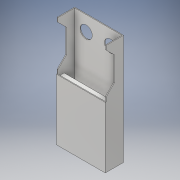
# Autodesk Inventor part: USB_Contact
Saved by Autodesk Inventor 2018 (Build 220112000, 112)
## iProperties
Created: 2018-02-01
Part Number: USB_Contact
Material: Generic
Document SubType Name: Modeling
Designer: Mandus
Density: 1 g/cm^3
Appearance: Default
Author: Mandus
Autodesk Inventor part; units mm, degrees
ref_plane "YZ Plane" through (0, 0, 0) normal (1, 0, 0) x (0, 1, 0)
ref_plane "XZ Plane" through (0, 0, 0) normal (0, 1, 0) x (-1, 0, 0)
ref_plane "XY Plane" through (0, 0, 0) normal (0, 0, 1) x (1, 0, 0)
sketch "Sketch1" plane through (0, 0, 0) normal (0, 1, 0) x (-1, 0, 0)
  line L0 (5.3848, 9.7652) -> (-6.6152, 9.7652)
  line L1 (-6.6152, 9.7652) -> (-6.6152, 5.2652)
  line L2 (-6.6152, 5.2652) -> (5.3848, 5.2652)
  line L3 (5.3848, 5.2652) -> (5.3848, 9.7652)
  point P0 (0, 0)
  dimension "d0" = 12
  dimension "d1" = 4.5
  constraints: 8 end point, 2 parallel, 1 horizontal, 1 perpendicular
  measures "d0" distance of L2.end L1.end
  measures "d1" distance of L1.end L0.end
extrude "Extrusion1" add sketch "Sketch1" along normal blind 27
shell "Shell1" thickness 0.2 removed faces 2 at (2.6152, 27, 8.2652) at (2.6152, 0, 8.2652)
sketch "Sketch2" plane through (6.6152, 0, 9.7652) normal (1, 0, 0) x (0, 0, -1)
  line L0 (0, 0) -> (0, 27) projected
  line L1 (0, 27) -> (0, 15)
  line L2 (0, 15) -> (0.2, 15)
  line L3 (0.2, 15) -> (0.2, 16)
  line L4 (0, 27) -> (0.2, 27)
  line L5 (0.2, 27) -> (0.2, 26)
  line L6 (0.2, 27) -> (4.3, 27) projected
  line L7 (0.2, 26) -> (2.25, 23.95)
  line L8 (0.2, 16) -> (2.25, 18.05)
  line L9 (2.25, 18.05) -> (2.25, 23.95)
  line L10 (0, 0) -> (0, 27) projected
  point P0 (9.7652, 0)
  dimension "d5" = 12
  dimension "d6" = 0.2
  dimension "d7" = 1
  dimension "d9" = 1
  dimension "d12" = 2.05
  dimension "d15" = 2.05
  dimension "d16" = 5.9
  dimension "d17" = 2.05
  constraints: 16 end point, 2 horizontal, 2 perpendicular, 1 parallel, 1 point on line
  measures "d5" distance of L0.end L1.end
  measures "d6" distance of L1.end L2.end
  measures "d7" distance of L2.end L3.end
  measures "d9" distance of L4.end L5.end
  measures "d12" horizontal distance of L7.end L5.end
  measures "d15" horizontal distance of L8.end L3.end
  measures "d16" distance of L8.end L7.end
  measures "d17" horizontal distance of L8.end L3.end
extrude "Extrusion2" cut sketch "Sketch2" against normal up to next
sketch "Sketch3" plane through (-5.1848, 0, 5.4652) normal (0, 0, 1) x (1, 0, 0)
  circle A0 centre (2.8, 23.3) radius 1.5
  circle A1 centre (8.8, 23.3) radius 1.5
  line L0 (0, 27) -> (11.6, 27) projected
  line L1 (-0.2, 23.95) -> (-0.2, 26) projected
  line L2 (11.8, 26) -> (11.8, 23.95) projected
  point P0 (5.1848, 0)
  dimension "d20" = 3
  dimension "d21" = 3.7
  dimension "d22" = 3
  dimension "d23" = 3
  constraints: 2 centre point, 1 equal radius, 1 horizontal alignment
  measures "d20" diameter of A0
  measures "d21" distance from line of L0 A0.centre
  measures "d22" distance from line of L1 A0.centre
  measures "d23" distance from line of L2 A1.centre
extrude "Extrusion3" cut sketch "Sketch3" against normal up to next
sketch "Sketch4" plane through (0, 0, 0) normal (0, -1, 0) x (1, 0, 0)
  line L0 (-5.1848, 9.5652) -> (-5.3848, 9.5652) projected
  line L1 (-5.1848, 9.5652) -> (6.4152, 9.5652)
  line L2 (6.4152, 9.5652) -> (6.4152, 8.0652)
  line L3 (6.4152, 8.0652) -> (-5.1848, 8.0652)
  line L4 (-5.1848, 8.0652) -> (-5.1848, 9.5652)
  point P0 (0, 0)
  dimension "d26" = 11.6
  dimension "d27" = 1.5
  constraints: 8 end point, 2 parallel, 1 horizontal, 1 perpendicular
  measures "d26" distance of L2.end L3.end
  measures "d27" distance of L1.end L2.end
extrude "Extrusion4" add sketch "Sketch4" along normal blind 1 and the other way blind 14.5
move faces "Move1" translate (0, 1.5, 0) faces at (-1.3181, -1, 9.0652)
body "Solid1"
